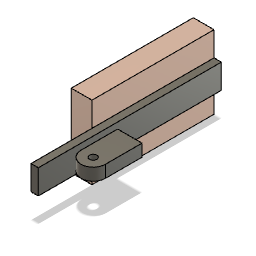
stamp pad 1 v3 (Autodesk Fusion 360 design; units mm, degrees)
Autodesk Fusion 360 part; units mm, degrees
sketch "Sketch1" plane through (0, 0, 0) normal (1, 0, 0) x (0, 0, -1)
  line L0 (-50, 30) -> (50, 30)
  line L1 (50, 30) -> (50, -30)
  line L2 (50, -30) -> (-50, -30)
  line L3 (-50, -30) -> (-50, 30)
  line L4 (48, -28) -> (-48, -28)
  line L5 (-48, -28) -> (-48, 28)
  line L6 (-48, 28) -> (48, 28)
  line L7 (48, 28) -> (48, -28)
  dimension "d1" = 100
  dimension "d2" = 60
  dimension "d3" = 2
  dimension "d17" = 30
  dimension "d18" = 50
  constraint horizontal L0
  constraint perpendicular L0 L1
  constraint parallel L0 L2
  constraint parallel L1 L3
  measures "d1" distance of L1.end L2.end
  measures "d2" distance of L0.end L1.end
  measures "d17" distance of L0 origin
  measures "d18" distance of origin L3
extrude "Extrude1" add sketch "Sketch1" along normal blind 2 contours L0 L1 L2 L3 | L4 L5 L6 L7 makes body 1
extrude "Extrude2" add sketch "Sketch1" against normal blind 15 bodies 1
sketch "Sketch2" plane through (0, 0, 0) normal (-1, 0, 0) x (0, 0, 1)
  line L0 (-48, 28) -> (-48, -28)
  line L1 (-48, -28) -> (48, -28)
  line L2 (48, -28) -> (48, 28)
  line L3 (48, 28) -> (-48, 28)
  line L4 (45, 25) -> (-45, 25)
  line L5 (-45, 25) -> (-45, -25)
  line L6 (-45, -25) -> (45, -25)
  line L7 (45, -25) -> (45, 25)
  line L8 (45, 25) -> (-45, -25) construction
  line L9 (-45, 25) -> (45, -25) construction
  dimension "d8" = 90
  dimension "d9" = 50
  constraint horizontal L4
  constraint perpendicular L4 L5
  constraint parallel L4 L6
  constraint parallel L5 L7
  constraint coincident L8 origin
  constraint coincident L9 origin
  measures "d8" distance of L5.end L6.end
  measures "d9" distance of L4.end L5.end
extrude "Extrude3" add sketch "Sketch2" along normal blind 13 contours L4 L5 L6 L7 bodies 1
sketch "Sketch4" plane through (2, 0, 0) normal (1, 0, 0) x (0, 0, -1)
  line L0 (-50, -30) -> (50, -30)
  line L1 (50, -30) -> (50, 30)
  line L2 (50, 30) -> (-50, 30)
  line L3 (-50, 30) -> (-50, -30)
  line L4 (50, -10) -> (-100, -10)
  line L5 (-100, -10) -> (-100, 10)
  line L6 (-100, 10) -> (50, 10)
  line L7 (50, 10) -> (50, -10)
  point P0 (-50, -10)
  point P1 (50, -10)
  dimension "d22" = 20
  constraint coincident L3 P0
  constraint horizontal L4
  constraint vertical L5
  constraint horizontal L6
  constraint vertical L7
  constraint coincident P1 L4.start
  measures "d22" distance of P1 L6.end
extrude "Extrude4" add sketch "Sketch4" along normal blind 6 contours L3 L4 L5 L6 | L1 L3 L4 L6 L7 bodies 1
sketch "Sketch5" plane through (0, -10, 0) normal (0, -1, 0) x (1, 0, 0)
  line L0 (2, 50) -> (2, -50)
  line L1 (2, -50) -> (8, -50)
  line L2 (8, -50) -> (8, 100)
  line L3 (8, 100) -> (2, 100)
  line L4 (2, 100) -> (2, 50)
  circle A0 centre (18, 65) radius 3
  line L5 (28, 65) -> (28, 35)
  line L6 (28, 35) -> (8, 35)
  arc A1 (28, 65) -> (8, 65) centre (18, 65) ccw
  dimension "d26" = 10
  dimension "d27" = 6
  constraint coincident L2 A1.end
  constraint concentric A0 A1
  constraint tangent L5 A1
  constraint parallel L2 L5
  constraint coincident L2 L6.end
  constraint perpendicular L2 L6
  measures "d26" distance of A1.end A0.centre
  measures "d27" diameter of A0
extrude "Extrude5" add sketch "Sketch5" against normal blind 10 from surface at -5 contours L2 L5 L6 A1 bodies 1
sketch "Sketch6" plane through (0, -30, 0) normal (0, -1, 0) x (1, 0, 0)
  line L0 (-15, -50) -> (2, -50)
  line L1 (2, -50) -> (2, 50)
  line L2 (2, 50) -> (-15, 50)
  line L3 (-15, 50) -> (-15, -50)
  line L4 (-3.4442, -44.9299) -> (-3.4442, 44.3486) construction
  line L5 (-3.4442, 44.3486) -> (-9.7091, 44.3486) construction
  line L6 (-9.7091, 44.3486) -> (-9.7091, -44.9299) construction
  line L7 (-9.7091, -44.9299) -> (-3.4442, -44.9299) construction
  dimension "d32" = 10
  text T0 "STAMP PAD" font "Arial" height 10 align centre middle in box 89.2785 x 6.2649 at (-3.4442, -44.9299) x (0, 1) y (-1, 0) spacing 1 kerned
emboss "Emboss2" depth -2 profiles "Sketch6" section 1 text T0 onto face at (-9.3333, -30, -16.6667) on bodies 1 bodies 1 makes body 2 at (-8.0137, -28, 2.4504) makes body 3 at (-6.6062, -30, 24.3399) makes body 4 at (-8.0137, -30, 15.3972) makes body 5 at (-6.6017, -28, 34.5536) makes body 6 at (-6.6062, -28, -17.8429)
